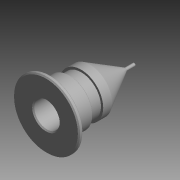
# Autodesk Inventor part: Nozzle
Saved by Autodesk Inventor 2015 (Build 190159000, 159)
## iProperties
Created: 2015-01-06
Part Number: Nozzle
Material: Generic
Document SubType Name: Modeling
Designer: ice
Density: 1 g/cm^3
Appearance: Default
Mass: 1.02114 g
Surface Area: 9.24729 cm^2
Volume: 1.02114 cm^3
Author: ice
Autodesk Inventor part; units mm, degrees
ref_plane "YZ Plane" through (0, 0, 0) normal (1, 0, 0) x (0, 1, 0)
ref_plane "XZ Plane" through (0, 0, 0) normal (0, 1, 0) x (-1, 0, 0)
ref_plane "XY Plane" through (0, 0, 0) normal (0, 0, 1) x (1, 0, 0)
sketch "Sketch1" plane through (0, 0, 0) normal (0, 0, 1) x (1, 0, 0)
  line L0 (0, 14.375) -> (0, 5.6)
  line L1 (0, 14.375) -> (0, 17.5)
  line L2 (-0.35, 17.5) -> (-0.35, 15.554)
  line L3 (0, 17.5) -> (0, 5.6)
  line L4 (-0.35, 17.5) -> (0, 17.5)
  line L5 (-5, 7.5) -> (-0.35, 15.554)
  line L6 (-5, 7.5) -> (6.0041, 7.5) construction
  line L7 (-5, -2.5) -> (-2.8, -2.5)
  line L8 (-2.8, -2.5) -> (0, -2.5)
  line L9 (0, -2.5) -> (0, 5.6)
  line L10 (-5, 7.5) -> (-5, 5.5)
  line L11 (-5, 5.5) -> (-4.5, 5.5)
  line L12 (-4.5, 5.5) -> (-4.5, 3)
  line L13 (-4.5, 3) -> (-5, 3)
  line L14 (-5, 7.5) -> (-5, 5.5)
  line L15 (-5, -2.5) -> (-7.5, -2.5)
  line L16 (-5.25, -0.5) -> (-5.25, 1.5)
  line L17 (-5, 3) -> (-5.25, 3)
  line L18 (-5.25, 3) -> (-5.25, 2.75)
  line L19 (-5.25, 2.75) -> (-5.25, 1.5)
  line L20 (-5.25, -0.5) -> (-5.25, -1.5)
  line L21 (-5.25, -1.5) -> (-7.5, -1.5)
  line L22 (-7.5, -1.5) -> (-7.5, -2.5)
  dimension "d81" = 60
  dimension "d82" = 10
  dimension "d83" = 0.35
  dimension "d84" = 1.946
  dimension "d85" = 8.054
  dimension "d87" = 10
  dimension "d106" = 20
  dimension "d107" = 5
  dimension "d131" = 2
  dimension "d132" = 0.5
  dimension "d133" = 2.5
  dimension "d134" = 2.5
  dimension "d138" = 0.25
  dimension "d139" = 0.25
  dimension "d144" = 4.5
  dimension "d145" = 1
  constraints: 46 end point, 7 perpendicular, 3 horizontal, 3 vertical, 2 collinear, 1 point on line
  measures "d81" angle of L6 L5
  measures "d82" vertical distance of L2.start L5.start
  measures "d83" distance of L2.start L1.end
  measures "d84" distance of L2.end L2.start
  measures "d85" vertical distance of L5.start L2.end
  measures "d87" distance of L5.start L7.start
  measures "d106" distance of L1.end L8.end
  measures "d107" distance of L8.end L7.start
  measures "d131" distance of L5.start L10.end
  measures "d132" distance of L10.end L11.end
  measures "d133" distance of L11.end L12.end
  measures "d134" distance of L7.start L15.end
  measures "d138" distance of L13.end L17.end
  measures "d139" distance of L17.end L18.end
  measures "d144" distance of L20.end L17.end
  measures "d145" distance of L21.end L15.end
revolve "Revolution1" add sketch "Sketch1" angle 360 about axis through (0, 14.375, 0) along (0, -1, 0)
ref_plane "Work Plane3" through (0, -2.5, 0) normal (0, 1, 0) x (-1, 0, 0)
sketch "Sketch5" plane through (0, -2.5, 0) normal (0, 1, 0) x (-1, 0, 0)
  point P0 (0, 0)
sketch "Sketch6" plane through (0, -2.5, 0) normal (0, -1, 0) x (1, 0, 0)
  circle A0 centre (0, 0) radius 2.9
  dimension "d108" = 5.8
  constraints: 1 centre point, 1 coincident
  measures "d108" diameter of A0
hole "Hole6" at (0, -2.5, 0) direction (0, 1, 0) diameter 5.8 depth 7.25 tip angle 118
hole "Hole7" at (0, -2.5, 0) direction (0, 1, 0) diameter 2 depth 15 tip angle 118
sketch "Sketch7" plane through (0, 17.5, 0) normal (0, 1, 0) x (1, 0, 0)
  circle A0 centre (0, 0) radius 0.075
  dimension "d123" = 0.15
  constraints: 1 centre point, 1 coincident
  measures "d123" diameter of A0
hole "Hole8" at (0, 17.5, 0) direction (0, -1, 0) diameter 0.3 end through all
chamfer "Chamfer1" distance 0.25 angle 45 4 edges at (5.25, 3, 0) (7.5, -2.5, 0) (0, -2.5, 2.9) (7.5, -1.5, 0)
body "Solid1"
